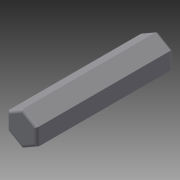
# Autodesk Inventor part: 000107-1
Saved by Autodesk Inventor 2015 (Build 190159000, 159)
## iProperties
Created: 2015-05-11
Part Number: 000107-1
Material: Generic
Document SubType Name: Modeling
Designer: Wesley
Density: 1 g/cm^3
Appearance: Default
Author: Wesley
Autodesk Inventor part; units mm, degrees
ref_plane "YZ Plane" through (0, 0, 0) normal (1, 0, 0) x (0, 1, 0)
ref_plane "XZ Plane" through (0, 0, 0) normal (0, 1, 0) x (-1, 0, 0)
ref_plane "XY Plane" through (0, 0, 0) normal (0, 0, 1) x (1, 0, 0)
sketch "Sketch1" plane through (0, 0, 0) normal (0, 0, 1) x (1, 0, 0)
  line L0 (0, 1.5875) -> (1.3748, 0.7937)
  line L1 (1.3748, 0.7937) -> (1.3748, -0.7937)
  line L2 (1.3748, -0.7937) -> (0, -1.5875)
  line L3 (0, -1.5875) -> (-1.3748, -0.7938)
  line L4 (-1.3748, -0.7938) -> (-1.3748, 0.7937)
  line L5 (-1.3748, 0.7937) -> (0, 1.5875)
  point P0 (0, 0)
  point P1 (0, 0)
  dimension "d0" = 3.175
  dimension "d6" = 1.3748
  constraints: 12 end point, 1 coincident, 13 other
  measures "d0" distance of L2.end L0.start
  measures "d6" horizontal distance of L1.end L2.end
extrude "Extrusion1" add sketch "Sketch1" along normal blind 12.7
fillet "Fillet1" radius 0.254 12 edges at (-0.6874, 1.1906, 12.7) (-1.3748, 0, 12.7) (-0.6874, -1.1906, 12.7) (0.6874, -1.1906, 12.7) (1.3748, 0, 12.7) (0.6874, 1.1906, 12.7) (-0.6874, 1.1906, 0) (0.6874, 1.1906, 0) (1.3748, 0, 0) (0.6874, -1.1906, 0) (-0.6874, -1.1906, 0) (-1.3748, 0, 0)
body "Solid1"
